m3_nut (Autodesk Fusion 360 design; units mm, degrees)
Autodesk Fusion 360 part; units mm, degrees
sketch "Sketch1" plane through (0, 0, 0) normal (1, 0, 0) x (0, 1, 0)
  line L0 (-1.53, 2.65) -> (1.53, 2.65)
  line L1 (1.53, 2.65) -> (3.06, 0)
  line L2 (3.06, 0) -> (1.53, -2.65)
  line L3 (1.53, -2.65) -> (-1.53, -2.65)
  line L4 (-1.53, -2.65) -> (-3.06, 0)
  line L5 (-3.06, 0) -> (-1.53, 2.65)
  line L6 (1.53, 2.65) -> (1.53, -2.65)
  line L7 (3.06, 0) -> (-3.06, 0)
  circle A0 centre (0, 0) radius 1.25
  dimension "d1" = 120
  dimension "d2" = 120
  dimension "d3" = 120
  dimension "d5" = 5.3
  dimension "d6" = 5.3
  dimension "d10" = 2.5
  constraint horizontal L0
  constraint parallel L0 L3
  constraint parallel L1 L4
  constraint midpoint A0.centre L7
  constraint perpendicular L6 L7
  constraint parallel L0 L7
  constraint coincident A0.centre origin
  measures "d1" angle of L0 L5
  measures "d2" angle of L0 L1
  measures "d3" angle of L1 L2
  measures "d5" distance of L0 L3
  measures "d6" distance of L1 L4
  measures "d10" diameter of A0
extrude "Extrude1" add sketch "Sketch1" along normal blind 2.2 contours L0 L5 L6 L7 A0 | L1 L6 L7 | L3 L4 L6 L7 A0 | L2 L6 L7
move_face "OffsetFaces1" offset 0.2 8 faces at (2.2, 0.0311, -2.1822) (1.4667, 2.55, 0.8833) (0.7333, 2.55, -0.8833) (0.7333, 0.51, -2.65) (1.4667, -2.55, -0.8833) (0.7333, -2.55, 0.8833) (0.7333, -0.51, 2.65) (0, 0.0311, -2.1822)
equation "d2 = d1"
equation "d3 = d1"
equation "d6 = d5"
